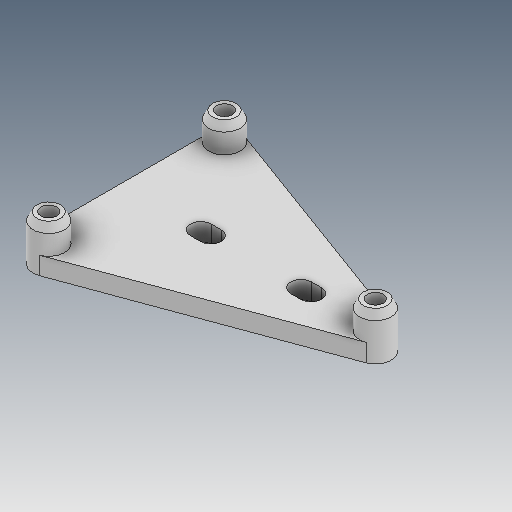
# Autodesk Inventor part: db-25_standoffs_plate_t-slot-2inx1in
Saved by Autodesk Inventor 2025.1 (Build 291241000, 241)
## iProperties
Created: 2026-06-20
Part Number: db-25_standoffs_plate_t-slot-2inx1in
Material: Generic
Document SubType Name: Modeling
Designer: Aiden
Density: 1 g/cm^3
Appearance: Default
Author: Aiden
Autodesk Inventor part; units mm, degrees
ref_plane "YZ Plane" through (0, 0, 0) normal (1, 0, 0) x (0, 1, 0)
ref_plane "XZ Plane" through (0, 0, 0) normal (0, 1, 0) x (-1, 0, 0)
ref_plane "XY Plane" through (0, 0, 0) normal (0, 0, 1) x (1, 0, 0)
sketch "Connector Hole Layout" plane through (0, 0, 0) normal (0, 1, 0) x (-1, 0, 0)
  circle A0 centre (42.948752, 7.963756) radius 1.6 construction
  circle A1 centre (-17.538767, 30.213756) radius 1.6 construction
  circle A2 centre (42.948752, 52.463756) radius 1.6 construction
  line L0 (42.948752, 7.963756) -> (42.948752, 52.463756) construction
  line L1 (41.447122, 51.91139) -> (-16.037138, 30.766122) construction
  point P0 (42.948752, 30.213756)
  dimension "d0" = 3.2
  dimension "d22" = 44.5
  dimension "d23" = 61.25
  constraints: 4 end point, 3 coincident, 1 centre point, 1 horizontal alignment, 1 midpoint, 1 vertical, 1 vertical alignment, 10 other
  measures "d0" diameter of A0
  measures "d22" distance of L0.start L0.end
sketch "Sketch8" plane through (0, 0, 0) normal (0, 1, 0) x (-1, 0, 0)
  circle A0 centre (42.948752, 7.963756) radius 1.6 construction
  circle A1 centre (42.948752, 52.463756) radius 1.6 construction
  circle A2 centre (-17.538767, 30.213756) radius 1.6 construction
  circle A3 centre (42.948752, 7.963756) radius 4
  point P0 (0, 0)
  dimension "d51" = 8
  constraints: 4 coincident, 1 centre point
  measures "d51" diameter of A3
sketch "Sketch8 outline for Extrusion5" plane through (0, 0, 0) normal (0, 1, 0) x (-1, 0, 0)
  circle A0 centre (42.948752, 7.963756) radius 4
extrude "Extrusion5" add sketch "Sketch8 outline for Extrusion5" along normal blind 7
sketch "Sketch9" plane through (-42.948752, 7, 7.963756) normal (0, 1, 0) x (1, 0, 0)
  point P0 (42.948752, 7.963756)
  point P1 (0, 0)
hole "Hole2" at (-42.948752, 7, 7.963756) direction (0, -1, 0) diameter 4 depth 5 tip angle 118
chamfer "Chamfer3" distance 1 distance2 2 1 edges at (-38.9488, 7, 7.9638) measured on face at (-46.2385, 7, 7.5643)
pattern_sketch "Sketch Driven Pattern1" from (-42.948752, 0, 7.963756) copies at (-42.948752, 0, 52.463756) at (17.538767, 0, 30.213756)
sketch "Sketch10" plane through (-42.948752, 0, 52.463756) normal (0, -1, 0) x (1, 0, 0)
  circle A0 centre (0, 0) radius 4
  line L0 (1.380915, 3.754074) -> (61.868435, -18.495926)
  circle A1 centre (60.487519, -22.25) radius 4
  line L1 (61.868435, -26.004074) -> (1.380915, -48.254074)
  circle A2 centre (0, -44.5) radius 4
  line L2 (-4, -44.5) -> (-4, 0)
  circle A3 centre (0, 0) radius 4
  circle A4 centre (0, -44.5) radius 4
  point P0 (42.948752, -52.463756)
  constraints: 6 end point, 6 point on circle, 5 tangent, 2 other
sketch "Sketch10 outline for Extrusion6" plane through (-42.948752, 0, 52.463756) normal (0, -1, 0) x (1, 0, 0)
  line L0 (-4, 0) -> (-4, -44.5)
  arc A0 (1.380915, 3.754074) -> (-4, 0) centre (0, 0) ccw
  line L1 (61.868435, -18.495926) -> (1.380915, 3.754074)
  arc A1 (61.868435, -26.004074) -> (61.868435, -18.495926) centre (60.487519, -22.25) ccw
  line L2 (1.380915, -48.254074) -> (61.868435, -26.004074)
  arc A2 (-4, -44.5) -> (1.380915, -48.254074) centre (0, -44.5) ccw
extrude "Extrusion6" add sketch "Sketch10 outline for Extrusion6" along normal blind 4.5
sketch "Sketch11" plane through (-42.948752, 0, 52.463756) normal (0, 1, 0) x (1, 0, 0)
  line L0 (-4, 48.5) -> (64.487519, 48.5) construction
  line L1 (64.487519, 48.5) -> (64.487519, -4) construction
  line L2 (64.487519, -4) -> (-4, -4) construction
  line L3 (-4, -4) -> (-4, 48.5) construction
  circle A0 centre (60.487519, 22.25) radius 4 construction
  circle A1 centre (0, 0) radius 4 construction
  circle A2 centre (0, 44.5) radius 4 construction
  line L4 (30.24376, 48.5) -> (30.24376, -4) construction
  line L5 (-4, 22.25) -> (64.487519, 22.25) construction
  line L6 (16.27376, 22.25) -> (18.81376, 22.25) construction
  line L7 (16.27376, 19.65) -> (18.81376, 19.65)
  line L8 (18.81376, 24.85) -> (16.27376, 24.85)
  arc A3 (16.27376, 24.85) -> (16.27376, 19.65) centre (16.27376, 22.25) ccw
  arc A4 (18.81376, 19.65) -> (18.81376, 24.85) centre (18.81376, 22.25) ccw
  line L9 (44.21376, 19.65) -> (41.67376, 19.65)
  line L10 (41.67376, 24.85) -> (44.21376, 24.85)
  arc A5 (44.21376, 19.65) -> (44.21376, 24.85) centre (44.21376, 22.25) ccw
  arc A6 (41.67376, 24.85) -> (41.67376, 19.65) centre (41.67376, 22.25) ccw
  point P0 (42.948752, 52.463756)
  point P1 (30.24376, 22.25)
  point P2 (30.24376, 22.25)
  point P3 (17.54376, 22.25)
  point P4 (17.54376, 24.85)
  point P5 (17.54376, 19.65)
  dimension "d66" = 11.43
  dimension "d67" = 13.97
  dimension "d68" = 5.2
  constraints: 24 end point, 9 midpoint, 8 point on circle, 7 tangent, 6 symmetric about line, 4 centre point, 3 parallel, 2 point on line, 1 collinear, 1 horizontal, 1 horizontal alignment, 1 perpendicular, 1 vertical, 3 other
  measures "d66" distance of point (30.244, 22.25) L6.end
  measures "d67" distance of point (30.244, 22.25) L6.start
  measures "d68" distance of point (17.544, 24.85) point (17.544, 19.65)
sketch "Sketch11 outline for Extrusion7" plane through (-42.948752, 0, 52.463756) normal (0, 1, 0) x (1, 0, 0)
  arc A0 (44.21376, 19.65) -> (44.21376, 24.85) centre (44.21376, 22.25) ccw
  line L0 (41.67376, 19.65) -> (44.21376, 19.65)
  arc A1 (41.67376, 24.85) -> (41.67376, 19.65) centre (41.67376, 22.25) ccw
  line L1 (44.21376, 24.85) -> (41.67376, 24.85)
  line L2 (16.27376, 19.65) -> (18.81376, 19.65)
  arc A2 (16.27376, 24.85) -> (16.27376, 19.65) centre (16.27376, 22.25) ccw
  line L3 (18.81376, 24.85) -> (16.27376, 24.85)
  arc A3 (18.81376, 19.65) -> (18.81376, 24.85) centre (18.81376, 22.25) ccw
extrude "Extrusion7" cut sketch "Sketch11 outline for Extrusion7" against normal blind 10
body "Solid2"
